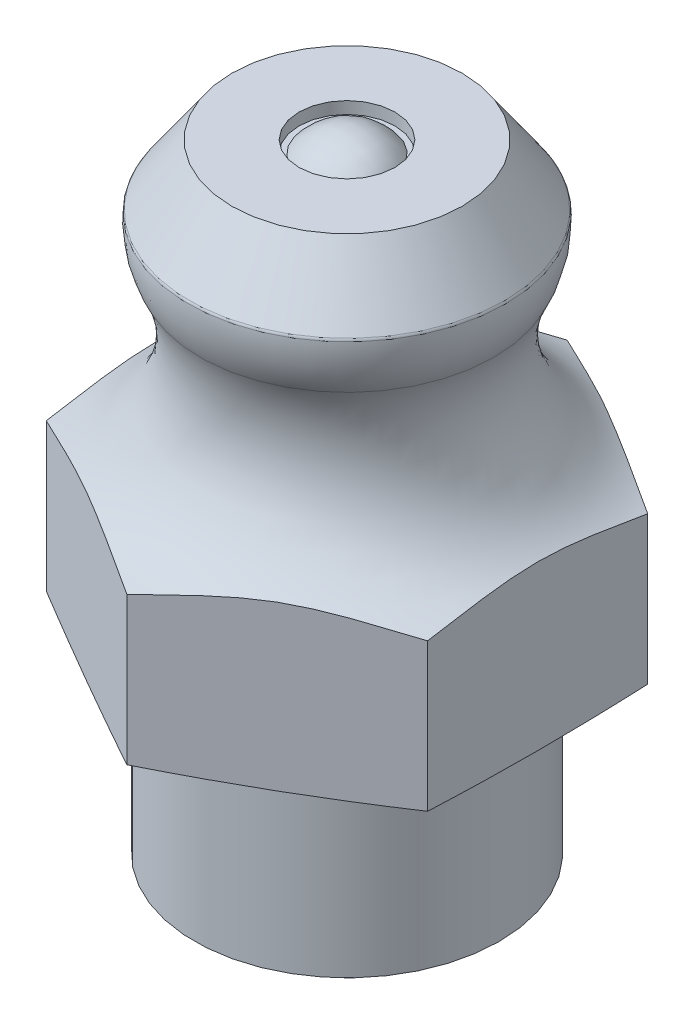
# Autodesk Inventor part: 1/4-28 UNF
Saved by Autodesk Inventor 2019 (Build 230136000, 136)
## iProperties
Created: 2024-04-15
Part Number: 1/4-28 UNF
Material: Generic
Catalog Web Link: www.cadenas.de
Description: 1/4-28 SAE-LT-Grease Nipple
Vendor: SKF
Document SubType Name: Modeling
Designer: psAdmin
Manufacturer: SKF
Mass: 0.376276 g
Surface Area: 5.28362 cm^2
Volume: 0.376276 cm^3
Density: 1 g/cm^3
Appearance: PSOLRGB-175-175-175
Category: PARTsolutions
Company: SKF
Title: 1/4-28 UNF
Author: Cadenas PARTsolutions
Comments: Grease Nipple
PSOL_IDENT_0: {$CADENAS_DATA/23d-libs/skf/bearings_units_and_housings/bearing_units/ball_bearing_units/y-unit_acce
PSOL_IDENT_1: ssories/grease_nipple.prj},167 {VTYP=3D},{NB=1/4-28 UNF},{LINA=1/4-28 UNF},{NN=1/4-28 SAE-LT},{DATE=
PSOL_IDENT_2: 21.11.2022 09:43:36},{GEOMDATE=29.07.2020 11:16:44},{VERSION=},{LINEID=30},{WBVAR=},{WBNUMERIC=}  {N
PSOL_IDENT_3: B=1/4-28 UNF},{LINA=1/4-28 UNF},{KT=DUMMY},{PN=1/4-28 UNF}
NB: 1/4-28 UNF
NN: 1/4-28 SAE-LT
NT: Grease Nipple
NBSYN: $PN.
LINA: 1/4-28 UNF
CATALOG: SKF
PN: 1/4-28 UNF
SUPPLIER: SKF
ARTICLENO: 1/4-28 UNF
BOMINFO: 1/4-28 UNF
CREATOR: CADENAS GmbH
Autodesk Inventor part; units mm, degrees
sketch "Sketch_4" plane through (0, 0, 0) normal (0, 0, 1) x (1, 0, 0)
  line L0 (0, -4.6) -> (0, 9.1)
  arc A0 (0.8874, 8.85) -> (0, 9.3) centre (0, 8.2) ccw
  line L1 (0.8874, 8.85) -> (1, 8.85)
  line L2 (1, 8.85) -> (1, 9.1)
  line L3 (1, 9.1) -> (2.4, 9.1)
  line L4 (2.4, 9.1) -> (3.283, 7.8389)
  arc A1 (3.3009, 7.788) -> (3.283, 7.8389) centre (3.2011, 7.7816) ccw
  arc A2 (3.0642, 6.7086) -> (3.3009, 7.788) centre (1.305, 7.66) ccw
  arc A3 (3.0642, 6.7086) -> (4.5779, 3.1966) centre (5.3, 5.59) ccw
  arc A4 (4.585, 3.187) -> (4.5779, 3.1966) centre (4.575, 3.187) ccw
  line L5 (4.585, 3.187) -> (4.585, 0.12)
  line L6 (4.585, 0.12) -> (3.175, -0.0034)
  line L7 (3.175, -0.0034) -> (3.175, -3.77)
  line L8 (3.175, -3.77) -> (2.605, -4.1)
  line L9 (2.605, -4.1) -> (2.005, -4.1)
  line L10 (2.005, -4.1) -> (2.005, -4.6)
  line L11 (2.005, -4.6) -> (1.305, -4.6)
  line L12 (1.305, -4.6) -> (1.305, -3.7)
  line L13 (1.305, -3.7) -> (1.5, -3.7)
  arc A5 (1.5, -3.7) -> (1.7, -3.5) centre (1.5, -3.5) ccw
  line L14 (1.7, -3.5) -> (1.7, 8.15)
  line L15 (1.7, 8.15) -> (1.1, 8.75)
  line L16 (1.1, 8.75) -> (0.9526, 8.75)
  arc A6 (0, 7.1) -> (0.9526, 8.75) centre (0, 8.2) ccw
  line L17 (0, 7.1) -> (0, 9.3)
  constraints: 36 end point, 14 point on circle, 7 centre point
revolve "Revolution1" add sketch "Sketch_4" angle 360 about axis through (0, -4.6, 0) along (0, -1, 0)
sketch "Sketch_5" plane through (0, 0, 0) normal (0, 1, 0) x (-1, 0, 0)
  line L0 (10, -10) -> (10, 10)
  line L1 (10, 10) -> (-10, 10)
  line L2 (-10, 10) -> (-10, -10)
  line L3 (-10, -10) -> (10, -10)
  line L4 (3.97, 2.2921) -> (0, 4.5842)
  line L5 (0, 4.5842) -> (-3.97, 2.2921)
  line L6 (-3.97, 2.2921) -> (-3.97, -2.2921)
  line L7 (-3.97, -2.2921) -> (0, -4.5842)
  line L8 (0, -4.5842) -> (3.97, -2.2921)
  line L9 (3.97, -2.2921) -> (3.97, 2.2921)
  constraints: 20 end point
extrude "Extrusion1" cut sketch "Sketch_5" along normal blind 5
ref_plane "gn_XY" through (0, 0, 0) normal (0, 0, 1) x (1, 0, 0)
ref_plane "gn_YZ" through (0, 0, 0) normal (1, 0, 0) x (0, 1, 0)
ref_plane "gn_ZX" through (0, 0, 0) normal (0, 1, 0) x (0, 0, 1)
body "Solid1"
